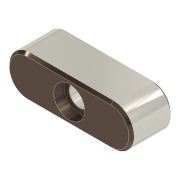
# Autodesk Inventor part: Slider
Saved by Autodesk Inventor 2022.2 (Build 262287010, 287A)
## iProperties
Created: 2022-12-29
Part Number: Slider
Material: Steel
Document SubType Name: Modeling
Designer: User
Mass: 10.0492 g
Surface Area: 8.67439 cm^2
Volume: 1.28016 cm^3
Density: 7.85 g/cm^3
Appearance: Gunmetal - Antique Polished
Author: User
Autodesk Inventor part; units mm, degrees
ref_plane "YZ Plane" through (0, 0, 0) normal (1, 0, 0) x (0, 1, 0)
ref_plane "XZ Plane" through (0, 0, 0) normal (0, 1, 0) x (-1, 0, 0)
ref_plane "XY Plane" through (0, 0, 0) normal (0, 0, 1) x (1, 0, 0)
sketch "Sketch1" plane through (0, 0, 0) normal (0, 0, 1) x (1, 0, 0)
  line L0 (-8, 0) -> (8, 0) construction
  line L1 (-8, -4) -> (8, -4)
  line L2 (8, 4) -> (-8, 4)
  arc A0 (-8, 4) -> (-8, -4) centre (-8, 0) ccw
  arc A1 (8, -4) -> (8, 4) centre (8, 0) ccw
  point P0 (0, 0)
  dimension "d0" = 16
  dimension "d1" = 4
  constraints: 8 end point, 4 point on circle, 4 tangent, 2 centre point, 1 horizontal, 1 midpoint, 1 parallel
  measures "d0" distance of L2.start L2.end
  measures "d1" radius of A1
extrude "Extrusion1" add sketch "Sketch1" along normal blind 8
chamfer "Chamfer1" distance 0.5 angle 45 8 edges at (0, 4, 8) (-12, 0, 8) (0, -4, 8) (12, 0, 8) (0, 4, 0) (-12, 0, 0) (0, -4, 0) (12, 0, 0)
sketch "Sketch2" plane through (0, 0, 8) normal (0, 0, 1) x (1, 0, 0)
  point P0 (0, 0)
hole "Hole1" at (0, 0, 8) direction (0, 0, -1) diameter 4 end through all counterbore diameter 6 counterbore depth 2
body "Solid1"
